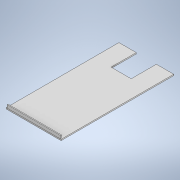
# Autodesk Inventor part: betonbottom
Saved by Autodesk Inventor 2021 (Build 250183000, 183)
## iProperties
Created: 2020-07-07
Part Number: betonbottom
Material: Generic
Document SubType Name: Modeling
Designer: adaml
Density: 1 g/cm^3
Appearance: Default
Author: adaml
Autodesk Inventor part; units mm, degrees
ref_plane "YZ Plane" through (0, 0, 0) normal (1, 0, 0) x (0, 1, 0)
ref_plane "XZ Plane" through (0, 0, 0) normal (0, 1, 0) x (-1, 0, 0)
ref_plane "XY Plane" through (0, 0, 0) normal (0, 0, 1) x (1, 0, 0)
sketch "Sketch1" plane through (0, 0, 0) normal (0, 0, 1) x (1, 0, 0)
  line L0 (0.222, 0) -> (0.222, -1)
  line L1 (0.222, 0) -> (0.222, -5.0532)
  line L2 (0.222, -1) -> (-0.778, -1)
  line L3 (-0.778, -1) -> (-0.778, -2.2)
  line L4 (53.594, 0) -> (55.372, 0)
  line L5 (53.594, 0) -> (53.594, -1)
  line L6 (53.594, 0) -> (53.594, -17.7031)
  line L7 (53.594, -1) -> (54.594, -1)
  line L8 (54.594, -1) -> (54.594, -2.2)
  line L9 (-1.778, 0) -> (-1.778, -17.5378)
  line L10 (-0.778, -2.2) -> (54.594, -2.2)
  line L11 (0.222, 0) -> (53.372, 0)
  line L12 (0.222, -1) -> (53.594, -1)
  line L13 (-0.778, -2.2) -> (54.594, -2.2)
  line L14 (54.594, -2.2) -> (54.594, -1)
  line L15 (54.594, -1) -> (-0.778, -1)
  line L16 (-0.778, -1) -> (-0.778, -2.2)
  line L17 (-0.278, -2.2) -> (-0.278, -1)
  line L18 (54.094, -2.2) -> (54.094, -1)
  point P0 (0, 0)
  point P1 (26.797, 5.3109)
  dimension "d0" = 1
  dimension "d1" = 1
  dimension "d2" = 1.2
  dimension "d3" = 1
  dimension "d4" = 1
  dimension "d5" = 1.2
  constraints: 38 end point, 7 perpendicular, 6 point on line, 2 parallel, 1 horizontal
  measures "d0" distance of L0.start L0.end
  measures "d1" distance of L0.end L2.end
  measures "d2" distance of L2.end L3.end
  measures "d3" distance of L4.start L5.end
  measures "d4" distance of L5.end L7.end
  measures "d5" distance of L7.end L8.end
extrude "Extrusion1" add sketch "Sketch1" along normal blind 111.76 contours L12 L6 L10 L1 | L1 L10 L17 L2 | L7 L18 L10 L6
sketch "Sketch2" plane through (-0.778, -1, 0) normal (0, 1, 0) x (1, 0, 0)
  line L0 (54.872, 0) -> (0.5, 0) projected
  line L1 (0, 0) -> (55.372, 0)
  line L2 (27.686, 0) -> (27.686, -25)
  line L3 (27.686, -25) -> (17.686, -25)
  line L4 (17.686, -25) -> (17.686, 0)
  line L5 (27.686, -25) -> (37.686, -25)
  line L6 (37.686, -25) -> (37.686, 0)
  line L7 (17.686, 0) -> (37.686, 0)
  point P0 (0.778, 0)
  dimension "d8" = 25
  dimension "d9" = 10
  dimension "d10" = 10
  constraints: 14 end point, 3 perpendicular, 3 point on line, 1 collinear, 1 horizontal, 1 midpoint, 1 vertical
  measures "d8" distance of L2.start L2.end
  measures "d9" distance of L2.end L3.end
  measures "d10" distance of L2.end L5.end
extrude "Extrusion2" cut sketch "Sketch2" against normal blind 111.76
sketch "Sketch3" plane through (-0.778, -1, 111.76) normal (0, 1, 0) x (1, 0, 0)
  line L0 (0, 111.76) -> (0, 0) projected
  line L1 (0, 0) -> (1.27, 0)
  line L2 (54.872, 0) -> (0.5, 0) projected
  line L3 (55.372, 0) -> (54.102, 0)
  line L4 (1.27, 0) -> (54.102, 0)
  line L5 (1.27, 0) -> (1.27, 0.9906)
  line L6 (1.27, 0.9906) -> (54.102, 0.9906)
  line L7 (54.102, 0.9906) -> (54.102, 0)
  point P0 (0.778, 111.76)
  dimension "d13" = 1.27
  dimension "d14" = 1.27
  dimension "d15" = 0.9906
  constraints: 12 end point, 2 point on line, 1 horizontal, 1 parallel, 1 perpendicular, 1 vertical
  measures "d13" distance of L0.end L1.end
  measures "d14" distance of L3.start L3.end
  measures "d15" distance of L1.end L5.end
ref_plane "Work Plane3" through (54.594, -1, 111.76) normal (0, -0.9957, 0.0929) x (-1, 0, 0)
ref_plane "Work Plane2" through (-0.778, -2.2, 111.76) normal (0, -0.0929, -0.9957) x (1, 0, 0)
sketch "Sketch5" plane through (54.594, -1, 111.76) normal (0, -0.9957, 0.0929) x (-1, 0, 0)
  line L0 (0, 111.76) -> (0, 0)
  line L1 (0, 0) -> (1.27, 0)
  line L2 (55.372, 0) -> (0, 0)
  line L3 (55.372, 0) -> (54.102, 0)
  line L4 (1.27, 0) -> (54.102, 0)
  line L5 (1.27, 0) -> (1.27, 0.9906)
  line L6 (1.27, 0.9906) -> (54.102, 0.9906)
  line L7 (54.102, 0.9906) -> (54.102, 0)
  point P0 (54.594, 111.1839)
  point P1 (0.778, 111.76)
  dimension "d26" = 1.27
  dimension "d27" = 1.27
  dimension "d28" = 0.9906
  constraints: 16 end point, 2 point on line, 1 horizontal, 1 parallel, 1 perpendicular, 1 vertical
  measures "d26" distance of L0.end L1.end
  measures "d27" distance of L2.start L3.end
  measures "d28" distance of L1.end L5.end
extrude "Extrusion5" add sketch "Sketch5" against normal blind 2.794
body "Solid1"
